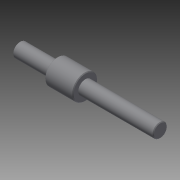
# Autodesk Inventor part: S1S 8L-1206_HUB0_0_0_0_0_SHNo_0__0_0__0_0__0_KEY_-_TAP1_0_0_0_0_0_TAP2_0_0_0_0_0
Saved by Autodesk Inventor 2014 SP2 (Build 180246200, 246)
## iProperties
Created: 2019-04-14
Part Number: S1S 8L-1206_HUB0_0_0_0_0_SHNo_0__0_0__0_0__0_KEY_-_TAP1_0_0_0_0_0_TAP2_0_0_0_0_0
Material: Generic
Catalog Web Link: www.cadenas.de
Description: Spur Gears-Module 1 (S45C, Shapes L1, L2)
Vendor: KYOUIKU
Document SubType Name: Modeling
Designer: psadmin
Manufacturer: KYOUIKU
Mass: 16.7 g
Surface Area: 14.6209 cm^2
Volume: 2.41156 cm^3
Density: 1 g/cm^3
Appearance: PSOLRGB-175-175-175
Category: PARTsolutions
Company: KYOUIKU
Title: S1S 8L-1206
Author: Cadenas PARTsolutions
Comments: Module 1 (S45C, Shapes L1, L2)
PSOL_IDENT_0: {$CADENAS_DATA\23d-libs\kyouiku\spur_gears\spur_gears_new_mod_1_s45c_l1_l2.prj},497 {VTYP=3D},{NB=S1
PSOL_IDENT_1: S 8L-1206_HUB0_0_0_0_0_SHNo_0__0_0__0_0__0_KEY_-_TAP1_0_0_0_0_0_TAP2_0_0_0_0_0},{LINA=S1S 8L-1206},{
PSOL_IDENT_2: NN=Spur Gears},{DATE=04.07.2018 06:05:09},{GEOMDATE=05.04.2018 11:13:15},{VERSION=},{LINEID=5560},{W
PSOL_IDENT_3: BVAR=HUB,HA,HB,HC,HD,SH,D1,TD1,DD1,D2,TD2,DD2,D3,TD3,DD3,KEY,TYPKEY,TAP1,NBTAP1,DTAP1,POSTAP1,ANGTAP
PSOL_IDENT_4: 01,ANGTAP1,TAP2,NBTAP2,DTAP2,POSTAP2,ANGTAP02,ANGTAP2},{WBNUMERIC=HUB,HA,HB,HC,HD,D1,DD1,D2,DD2,D3,D
PSOL_IDENT_5: D3,NBTAP1,DTAP1,POSTAP1,ANGTAP01,ANGTAP1,NBTAP2,DTAP2,POSTAP2,ANGTAP02,ANGTAP2}  {NB=S1S 8L-1206_HUB
PSOL_IDENT_6: 0_0_0_0_0_SHNo_0__0_0__0_0__0_KEY_-_TAP1_0_0_0_0_0_TAP2_0_0_0_0_0},{LINA=S1S 8L-1206},{KT=DUMMY},{ID
PSOL_IDENT_7: NR=},{CNSORDERNO=S1S 8L-1206},{X=0},{SSS=-},{MOD=1.00},{MTR=S45C},{Z=8},{D=8.0},{DA=10.6},{S=L1},{DB
PSOL_IDENT_8: 1=0},{B=12.0},{DD=0},{DH=6.0},{BXH=-},{LH=16.0},{LHR=32.00},{L=60.0},{B2=0.0},{T2=0.0},{NDM=0.0},{M=
PSOL_IDENT_9: -},{LS=0.0},{DI=0.0},{BW=0},{SP1=8},{FTS=-},{SP3=20},{SP6=+0.5},{SP7=2},{SP8=4.882},{MASS=16.70},{MS
PSOL_IDENT_10: X=16.70},{H1=0.00},{H2=0.00},{L1=0},{H3=0.00},{L2=0.00},{R=0.0000},{DB=0},{R1=16.00},{ON=S1S 8L-1206
PSOL_IDENT_11: },{VERS=0},{VERS2=1},{VERS1=1},{MX=1},{HUB=0},{XHUB=0,'No','hub_0.jpg'},{HA=0.00},{XHA=0},{HB=0.0},{
PSOL_IDENT_12: XHB=0},{HC=0.00},{XHC=0},{HD=0.0},{XHD=0},{HE=0},{HAMIN=0.10},{HAMAX=6},{HBMIN=0.0},{HBMAX=16.0},{HC
PSOL_IDENT_13: MIN=0.00},{HCMAX=-0.10},{HDMIN=0.1},{HDMIN2=17.0},{HDMAX=0.0},{HDMAX2=-0.1},{HCX=-0.05},{HDX=0.1},{L
PSOL_IDENT_14: HB=28},{DF=5.5},{SH=No},{XSH='No','No','sh_no.jpg'},{D1=0.00},{XD1=<0>},{D1MIN=0.00},{D1MAX=0.00},{T
PSOL_IDENT_15: D1=},{XTD1='','-'},{DD1=0.0},{XDD1=<0>},{DD1MIN=0.0},{DD1MIN2=0.0},{DD1MAX=0.0},{DD1MAX2=0.0},{D2=0.
PSOL_IDENT_16: 00},{XD2=<0>},{D2MIN=0.00},{D2MAX=0.00},{TD2=},{XTD2='','-'},{DD2=0.0},{XDD2=<0>},{DD2MIN=0.0},{DD2M
PSOL_IDENT_17: AX=28.0},{DD2MAX2=0.0},{DD2MIN2=0.0},{D3=0.00},{XD3=<0>},{D3MIN=0.00},{D3MAX=0.00},{TD3=},{XTD3='','
PSOL_IDENT_18: -'},{DD3=0.0},{XDD3=<0>},{DD3MIN=0.0},{DD3MAX=28.0},{D1X=0},{D2X=0},{D3X=0},{DD1X=0},{DD2X=14},{D2S=
PSOL_IDENT_19: 0},{D3S=0},{DD1S=6},{DD2S=12},{DDX=0},{KEY=},{TYPKEY=-},{XKEY=<'','-'>},{XTYPKEY='-','-'},{DKEY=0},{
PSOL_IDENT_20: DKEYMAX=4.8},{T2MIN=1},{BMIN=2},{DKEYMIN=2.828427},{B2X=0},{T2X=0},{DKEYMAX2=0},{TAP1=},{XTAP1='','-'
PSOL_IDENT_21: },{XTAP1X='','-'},{NBTAP1=0},{XNBTAP1=0,'-'},{DTAP1=0},{XDTAP=0,'-'},{POSTAP1=0.0},{XPOSTAP=0},{XPOS
PSOL_IDENT_22: TAPX1=0},{XPOSTAP2=0},{ANGTAP01=0},{ANGTAP1=0},{TAP2=},{XTAP2='','-'},{NBTAP2=0},{XNBTAP2=0,'-'},{DT
PSOL_IDENT_23: AP2=0},{XDTAP2=0,'-'},{TT1=0},{TT2=0},{TT3=0},{TT4=0},{DTAPMAX=0},{DTAPMAX1X=0},{DTAPMAX2=0},{DTAPMI
PSOL_IDENT_24: D=0},{DTAPMID1=0},{DTAPMID2=0},{DTAPTT1MAX=0},{DTAPTT1MAX2=0},{DTAPTT2MAX=0},{DTAPTT2MAX2=0},{DTAPTT
PSOL_IDENT_25: 3MAX=0},{DTAPTT3MAX2=0},{DTAPTT4MAX2=0},{POSTAPMIN=0.0},{POSTAPMIN2=0.0},{POSTAPMAX=15.0},{POSTAPMAX
PSOL_IDENT_26: 2=0.0},{POSMAX1=-1.0},{POSMAX2=-1.0},{POSMIN1=1.0},{POSMIN2=1.0},{XANGTAP01=0,'-'},{XANGTAP1=0,'-'},
PSOL_IDENT_27: {T2XX=0},{PMAX1=-1},{PMAX2=-1},{PMIN1=1},{PMIN2=1},{PMAX1X=-1},{PMAX2X=-1},{PMAX3X=-1},{PMIN1X=1},{P
PSOL_IDENT_28: MIN2X=1},{PMIN3X=1},{POSTAP2=0.0},{ANGTAP02=0},{ANGTAP2=0},{XANGTAP02=0,'-'},{XANGTAP2=0,'-'},{XDDX=
PSOL_IDENT_29: 0},{XDDX2=0},{XDHX=6},{XLX=60},{XLX2=0},{XT1X=0},{XT2X=0},{HAX=6},{SHX=No},{C1X=0.000},{C2X=0.3},{D1
PSOL_IDENT_30: MIN1=-1.5},{CNSORDERNOX=S1S 8L-1206_HUB0_0_0_0_0_SHNo_0__0_0__0_0__0_KEY_-_TAP1_0_0_0_0_0_TAP2_0_0_0
PSOL_IDENT_31: _0_0},{CNSORDERNO2=S1S 8L-1206_HUB0_0_0_0_0_SHNo_0__0_0__0_0__0_KEY_-_TAP1_0_0_0_0_0_TAP2_0_0_0_0_0}
PSOL_IDENT_32: ,{MZMS=19.000},{DIST=2.65},{TAPH=},{SP10=NA},{SP11=NA},{SP12=NA},{SP13=NA},{SP14=AV}
NN: Spur Gears
NT: Module 1 (S45C, Shapes L1, L2)
NB: S1S 8L-1206_HUB0_0_0_0_0_SHNo_0__0_0__0_0__0_KEY_-_TAP1_0_0_0_0_0_TAP2_0_0_0_0_0
NBSYN: $CNSORDERNOX.
LINA: S1S 8L-1206
CNSORDERNO: S1S 8L-1206
MOD: 1
MTR: S45C
Z: 8
D: 8
DA: 10.6
S: L1
B: 12
DD: 0
DH: 6
LH: 16
LHR: 32
L: 60
B2: 0
T2: 0
M: -
LS: 0
DI: 0
BW: 0
MASS: 16.70
HUB: 0
HA: 0
HB: 0
HC: 0
HD: 0
SH: Standard dimension
D1: 0
TD1: -
DD1: 0
D2: 0
TD2: -
DD2: 0
D3: 0
TD3: -
DD3: 0
KEY: -
TYPKEY: -
TAP1: -
NBTAP1: 0
DTAP1: 0
POSTAP1: 0
ANGTAP01: 0
ANGTAP1: 0
TAP2: -
NBTAP2: 0
DTAP2: 0
POSTAP2: 0
ANGTAP02: 0
ANGTAP2: 0
CNSORDERNO2: S1S 8L-1206_HUB0_0_0_0_0_SHNo_0__0_0__0_0__0_KEY_-_TAP1_0_0_0_0_0_TAP2_0_0_0_0_0
SUPPLIER: KYOUIKU
ARTICLENO: S1S 8L-1206_HUB0_0_0_0_0_SHNo_0__0_0__0_0__0_KEY_-_TAP1_0_0_0_0_0_TAP2_0_0_0_0_0
BOMINFO: S1S 8L-1206
CREATOR: CADENAS GmbH
Autodesk Inventor part; units mm, degrees
ref_plane "YZ Plane" through (0, 0, 0) normal (1, 0, 0) x (0, 1, 0)
ref_plane "XZ Plane" through (0, 0, 0) normal (0, 1, 0) x (-1, 0, 0)
ref_plane "XY Plane" through (0, 0, 0) normal (0, 0, 1) x (1, 0, 0)
sketch "Sketch_10" plane through (0, 0, 0) normal (0, 0, 1) x (1, 0, 0)
  line L0 (60, 0) -> (0, 0)
  line L1 (0, 0) -> (0, 2.7)
  line L2 (0, 2.7) -> (0.3, 3)
  line L3 (0.3, 3) -> (16, 3)
  line L4 (16, 3) -> (16, 5)
  line L5 (16, 5) -> (16.3, 5.3)
  line L6 (16.3, 5.3) -> (27.7, 5.3)
  line L7 (27.7, 5.3) -> (28, 5)
  line L8 (28, 5) -> (28, 3)
  line L9 (28, 3) -> (59.7, 3)
  line L10 (59.7, 3) -> (60, 2.7)
  line L11 (60, 2.7) -> (60, 0)
  line L12 (60, 0) -> (0, 0)
  constraints: 26 end point
revolve "Revolution1" add sketch "Sketch_10" angle 360 about axis through (60, 0, 0) along (1, 0, 0)
body "Solid1"
